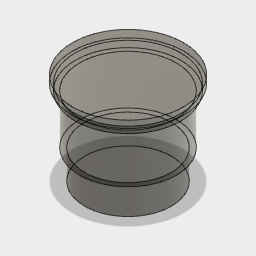
ボタン v0 (Autodesk Fusion 360 design; units mm, degrees)
Autodesk Fusion 360 part; units mm, degrees
sketch "スケッチ1" plane through (0, 0, 0) normal (0, 1, 0) x (1, 0, 0)
  circle A0 centre (0, 0) radius 14.8
  dimension "d1" = 29.6
  measures "d1" diameter of A0
extrude "押し出し1" add sketch "スケッチ1" along normal blind 10
sketch "スケッチ2" plane through (0, 10, 0) normal (0, 1, 0) x (-1, 0, 0)
  circle A0 centre (0, 0) radius 14.8
  circle A1 centre (0, 0) radius 16.5
  dimension "d4" = 33
  measures "d4" diameter of A1
extrude "押し出し2" add sketch "スケッチ2" along normal blind 19 contours A0 | A1
ref_plane "作業平面1" through (0, 24, 0) normal (0, 1, 0) x (-1, 0, 0)
sketch "スケッチ3" plane through (0, 24, 0) normal (0, 1, 0) x (1, 0, 0)
ref_plane "作業平面2" through (0, 29, 0) normal (0, -1, 0) x (-1, 0, 0)
sketch "スケッチ5" plane through (0, 29, 0) normal (0, -1, 0) x (1, 0, 0)
  circle A0 centre (0, 0) radius 19
  dimension "d12" = 38
  measures "d12" diameter of A0
extrude "押し出し4" add sketch "スケッチ5" against normal blind 2.5
sketch "スケッチ6" plane through (0, 29, 0) normal (0, -1, 0) x (1, 0, 0)
  circle A0 centre (0, 0) radius 18
  dimension "d15" = 36
  measures "d15" diameter of A0
extrude "押し出し5" add sketch "スケッチ6" along normal blind 2.2
ref_plane "作業平面4" through (0, 24.8, 0) normal (0, -1, 0) x (1, 0, 0)
